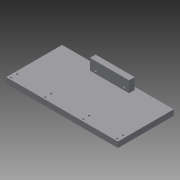
# Autodesk Inventor part: motor holder
Saved by Autodesk Inventor 2015 (Build 190159000, 159)
## iProperties
Created: 2014-10-18
Part Number: motor holder
Material: Generic
Document SubType Name: Modeling
Designer: ericd_000
Density: 1 g/cm^3
Appearance: Default
Author: ericd_000
Autodesk Inventor part; units mm, degrees
ref_plane "YZ Plane" through (0, 0, 0) normal (1, 0, 0) x (0, 1, 0)
ref_plane "XZ Plane" through (0, 0, 0) normal (0, 1, 0) x (-1, 0, 0)
ref_plane "XY Plane" through (0, 0, 0) normal (0, 0, 1) x (1, 0, 0)
sketch "Sketch1" plane through (0, 0, 0) normal (0, 0, 1) x (1, 0, 0)
  line L0 (-100, 50) -> (100, 50)
  line L1 (100, 50) -> (100, -50)
  line L2 (100, -50) -> (-100, -50)
  line L3 (-100, -50) -> (-100, 50)
  point P0 (0, 0)
  point P1 (100, 0)
  point P2 (0, 50)
  dimension "d0" = 200
  dimension "d1" = 100
  constraints: 8 end point, 2 midpoint, 2 parallel, 1 horizontal, 1 horizontal alignment, 1 perpendicular, 1 vertical alignment
  measures "d0" distance of L0.start L0.end
  measures "d1" distance of L2.end L0.start
extrude "Extrusion1" add sketch "Sketch1" along normal blind 10
sketch "Sketch2" plane through (0, 0, 10) normal (0, 0, 1) x (1, 0, 0)
  line L0 (30.48, -9.53) -> (-30.48, -9.53)
  line L1 (-30.48, -9.53) -> (-30.48, 40)
  line L2 (-30.48, 40) -> (30.48, 40)
  line L3 (30.48, 40) -> (30.48, -9.53)
  circle A0 centre (25.4, 34.92) radius 2.15
  line L4 (100, 50) -> (-100, 50) projected
  circle A1 centre (25.4, -4.45) radius 2.15
  circle A2 centre (-25.4, -4.45) radius 2.15
  circle A3 centre (-25.4, 34.92) radius 2.15
  point P0 (0, 0)
  point P1 (0, -9.53)
  dimension "d4" = 60.96
  dimension "d5" = 49.53
  dimension "d6" = 4.3
  dimension "d7" = 5.08
  dimension "d8" = 5.08
  dimension "d9" = 10
  dimension "d10" = 5.08
  dimension "d11" = 5.08
  dimension "d12" = 4.3
  dimension "d13" = 4.3
  dimension "d14" = 5.08
  dimension "d15" = 5.08
  dimension "d16" = 5.08
  dimension "d17" = 5.08
  dimension "d18" = 4.3
  constraints: 8 end point, 4 centre point, 2 parallel, 1 horizontal, 1 midpoint, 1 perpendicular, 1 vertical alignment
  measures "d4" distance of L0.start L0.end
  measures "d5" distance of L0.end L1.end
  measures "d6" diameter of A0
  measures "d7" distance from line of A0.centre L2
  measures "d8" distance from line of A0.centre L3
  measures "d9" distance between parallel lines of L4 L2
  measures "d10" distance from line of L0 A1.centre
  measures "d11" distance from line of A1.centre L3
  measures "d12" diameter of A1
  measures "d13" diameter of A2
  measures "d14" distance from line of L1 A2.centre
  measures "d15" distance from line of L0 A2.centre
  measures "d16" distance from line of L1 A3.centre
  measures "d17" distance from line of L2 A3.centre
  measures "d18" diameter of A3
extrude "Extrusion2" [suppressed]
sketch "Sketch3" plane through (0, 0, 10) normal (0, 0, 1) x (1, 0, 0)
  line L0 (98, -48) -> (28, -48)
  line L1 (28, -48) -> (28, -23)
  line L2 (28, -23) -> (98, -23)
  line L3 (98, -23) -> (98, -48)
  line L4 (-100, -50) -> (100, -50) projected
  line L5 (-100, 50) -> (-100, -50) projected
  line L6 (100, -50) -> (100, 50) projected
  circle A0 centre (95, -46) radius 1.4
  circle A1 centre (95, -35.5) radius 1.4
  circle A2 centre (34, -46) radius 1.4
  circle A3 centre (34, -35.5) radius 1.4
  line L7 (0, 0) -> (0, -50) construction
  circle A4 centre (-95, -46) radius 1.4
  circle A5 centre (-95, -35.5) radius 1.4
  circle A6 centre (-34, -46) radius 1.4
  circle A7 centre (-34, -35.5) radius 1.4
  dimension "d21" = 70
  dimension "d22" = 25
  dimension "d25" = 2
  dimension "d27" = 2
  dimension "d28" = 2.8
  dimension "d31" = 2.8
  dimension "d38" = 2.8
  dimension "d39" = 2.8
  dimension "d42" = 10.5
  dimension "d43" = 10.5
  dimension "d44" = 61
  dimension "d45" = 3
  dimension "d49" = 4
  constraints: 10 end point, 8 centre point, 4 symmetric about line, 2 parallel, 2 vertical alignment, 1 horizontal, 1 midpoint, 1 perpendicular, 4 other
  measures "d21" distance of L0.start L0.end
  measures "d22" distance of L0.end L1.end
  measures "d25" distance between parallel lines of L4 L0
  measures "d27" distance between parallel lines of L6 L3
  measures "d28" diameter of A0
  measures "d31" diameter of A1
  measures "d38" diameter of A3
  measures "d39" diameter of A2
  measures "d42" distance of A1.centre A0.centre
  measures "d43" distance of A2.centre A3.centre
  measures "d44" distance of A2.centre A0.centre
  measures "d45" distance from line of L3 A0.centre
  measures "d49" distance from line of L4 A0.centre
extrude "Extrusion4" cut sketch "Sketch3" against normal up to surface (10 mm away) contours A0 | A1 | A2 | A3 | A4 | A5 | A6 | A7
sketch "Sketch4" plane through (0, 0, 10) normal (0, 0, 1) x (1, 0, 0)
  line L0 (35, 35) -> (-35, 35)
  line L1 (-35, 35) -> (-35, 45)
  line L2 (-35, 45) -> (35, 45)
  line L3 (35, 45) -> (35, 35)
  line L4 (-100, -50) -> (100, -50) projected
  point P0 (0, 0)
  point P1 (0, 35)
  dimension "d50" = 85
  dimension "d51" = 10
  dimension "d52" = 70
  constraints: 8 end point, 2 parallel, 1 horizontal, 1 midpoint, 1 perpendicular, 1 vertical alignment
  measures "d50" distance between parallel lines of L4 L0
  measures "d51" distance of L2.end L0.start
  measures "d52" distance of L0.start L0.end
extrude "Extrusion5" add sketch "Sketch4" along normal blind 20
sketch "Sketch5" plane through (-100, 50, 0) normal (0, 1, 0) x (1, 0, 0)
  line L0 (130.48, -30.7809) -> (69.52, -30.7809)
  line L1 (69.52, -30.7809) -> (69.52, -15.7809)
  line L2 (69.52, -15.7809) -> (130.48, -15.7809)
  line L3 (130.48, -15.7809) -> (130.48, -30.7809)
  line L4 (0, 0) -> (200, 0) projected
  circle A0 centre (125.4, -15.1) radius 2.15
  circle A1 centre (74.6, -15.1) radius 2.15
  line L5 (200, -10) -> (135, -10) projected
  line L6 (65, -10) -> (0, -10) projected
  point P0 (100, 0)
  point P1 (100, 0)
  point P2 (100, -30.7809)
  dimension "d55" = 60.96
  dimension "d56" = 15
  dimension "d57" = 4.3
  dimension "d58" = 4.3
  dimension "d59" = 5.1
  dimension "d60" = 5.1
  dimension "d61" = 5.08
  dimension "d62" = 5.08
  constraints: 8 end point, 2 centre point, 2 midpoint, 2 parallel, 1 horizontal, 1 perpendicular, 1 vertical alignment
  measures "d55" distance of L0.start L0.end
  measures "d56" distance of L2.end L0.start
  measures "d57" diameter of A0
  measures "d58" diameter of A1
  measures "d59" distance from line of A0.centre L5
  measures "d60" distance from line of A1.centre L6
  measures "d61" distance from line of L1 A1.centre
  measures "d62" distance from line of L3 A0.centre
extrude "Extrusion6" cut sketch "Sketch5" against normal up to surface (15 mm away) contours A0 L2 | L2 A0 | A1 L2 | L2 A1
body "Solid1"
